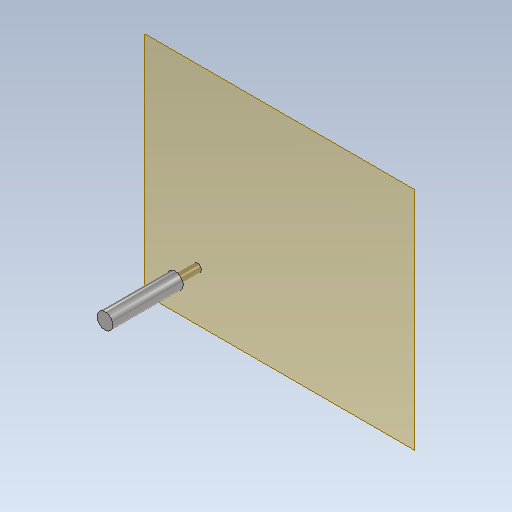
# Autodesk Inventor part: standoff
Saved by Autodesk Inventor 2020 (Build 240168000, 168)
## iProperties
Created: 2019-06-14
Part Number: standoff
Material: Stainless Steel
Document SubType Name: Modeling
Designer: amirt
Density: 8 g/cm^3
Appearance: Semi-Polished
Author: amirt
Autodesk Inventor part; units mm, degrees
ref_plane "YZ Plane" through (0, 0, 0) normal (1, 0, 0) x (0, 1, 0)
ref_plane "XZ Plane" through (0, 0, 0) normal (0, 1, 0) x (-1, 0, 0)
ref_plane "XY Plane" through (0, 0, 0) normal (0, 0, 1) x (1, 0, 0)
ref_plane "Work Plane1" through (0, 0, 0) normal (0, 0, 1) x (1, 0, 0)
sketch "Sketch1" plane through (0, 0, 0) normal (0, 0, 1) x (1, 0, 0)
  circle A0 centre (-29.8289, -24.3423) radius 1.1 projected
  point P0 (0, 0)
extrude "Extrusion1" add sketch "Sketch1" against normal blind 6.35
ref_plane "Work Plane2" through (0, 0, 0) normal (0, 0, 1) x (1, 0, 0)
sketch "Sketch2" plane through (0, 0, 0) normal (0, 0, 1) x (1, 0, 0)
  circle A0 centre (-29.8289, -24.3423) radius 1.1 projected
  circle A1 centre (-29.8289, -24.3423) radius 2.25
  point P0 (0, 0)
  dimension "d5" = 4.5
  constraints: 1 centre point, 1 coincident
  measures "d5" diameter of A1
extrude "Extrusion3" add sketch "Sketch2" along normal blind 20 contours A0 | A1
body "Solid1"
